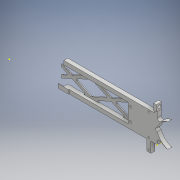
# Autodesk Inventor part: mtv_frame(BrakeInFront)2-6
Saved by Autodesk Inventor 2018 (Build 220112000, 112)
## iProperties
Created: 2019-01-13
Part Number: mtv_frame(BrakeInFront)2-6
Material: Generic
Document SubType Name: Modeling
Designer: aditya
Density: 1 g/cm^3
Appearance: Default
Author: aditya
## iProperties of the stored document mtv_frame(BrakeInFront)1-18 - FRONT_3DPrint.ipt
Created: 2019-01-19
Part Number: mtv_frame(BrakeInFront)1-18 - FRONT_3DPrint
Material: Generic
Document SubType Name: Modeling
Designer: aditya
Density: 1 g/cm^3
Appearance: Default
Author: aditya
Autodesk Inventor part; units mm, degrees
ref_plane "YZ Plane" through (0, 0, 0) normal (1, 0, 0) x (0, 1, 0)
ref_plane "XZ Plane" through (0, 0, 0) normal (0, 1, 0) x (-1, 0, 0)
ref_plane "XY Plane" through (0, 0, 0) normal (0, 0, 1) x (1, 0, 0)
sketch "Sketch1" plane through (0, 0, 0) normal (0, 1, 0) x (-1, 0, 0)
  line L0 (0, 0) -> (50, 0)
  line L1 (50, 0) -> (50, 50)
  line L2 (50, 50) -> (0, 50)
  line L3 (0, 50) -> (0, 0)
  line L4 (50, 50) -> (290, 50)
  line L5 (290, 50) -> (290, 42.5)
  line L6 (290, 42.5) -> (50, 42.5)
  line L7 (50, 42.5) -> (50, 50)
  line L8 (50, 0) -> (290, 0)
  line L9 (290, 0) -> (290, 7.5)
  line L10 (290, 7.5) -> (50, 7.5)
  line L11 (50, 7.5) -> (50, 0)
  dimension "d0" = 50
  dimension "d1" = 50
  dimension "d2" = 240
  dimension "d3" = 7.5
  dimension "d4" = 7.5
  constraints: 24 end point, 6 parallel, 3 horizontal, 3 perpendicular, 1 point on line
  measures "d0" distance of L2.end L1.end
  measures "d1" distance of L1.end L0.end
  measures "d2" distance of L5.end L6.end
  measures "d3" distance of L4.end L5.end
  measures "d4" distance of L9.end L8.end
extrude "Extrusion1" add sketch "Sketch1" along normal blind 7.5
sketch "Sketch2" plane through (0, 7.5, 0) normal (0, 1, 0) x (1, 0, 0)
  line L0 (0, -50) -> (0, 0) projected
  point P0 (0, -25)
  constraints: 1 midpoint
hole "Hole1" at (0, 7.5, 25) direction (0, -1, 0) diameter 6.35 end through all
sketch "Sketch3" plane through (0, 7.5, 0) normal (0, 1, 0) x (1, 0, 0)
  line L0 (-3.175, -50) -> (-3.175, 0) construction
  line L1 (-3.175, -50) -> (-28.175, -50) construction
  line L2 (-28.175, -50) -> (-28.175, 0) construction
  line L3 (-28.175, 0) -> (-3.175, 0) construction
  point P0 (0, 0)
  point P1 (-7.175, -4)
  point P2 (-24.175, -46)
  dimension "d14" = 25
  constraints: 8 end point, 2 perpendicular, 1 vertical
  measures "d14" distance of L0.start L1.end
hole "Hole2" at (-7.175, 7.5, 4) at (-24.175, 7.5, 46) direction (0, -1, 0) diameter 3.3 end through all
sketch "Sketch4" plane through (0, 7.5, 0) normal (0, 1, 0) x (1, 0, 0)
  arc A0 (0, -21.825) -> (0, -28.175) centre (0, -25) ccw construction
  line L0 (-3.175, -25) -> (-28.175, -25) construction
  line L1 (-3.175, -25) -> (21.825, -25) construction
  line L2 (-290, -50) -> (0, -50) construction
  line L3 (-28.175, -50) -> (-28.175, 0) construction
  line L4 (-50, -7.5) -> (-50, -42.5) construction
  line L5 (-50, -42.5) -> (-45, -42.5) construction
  line L6 (-45, -42.5) -> (-45, -32.5) construction
  line L7 (-45, -32.5) -> (-50, -32.5) construction
  line L8 (-50, -32.5) -> (-50, -42.5) construction
  line L9 (-45, -32.5) -> (-40, -32.5)
  line L10 (-40, -32.5) -> (-40, -42.5)
  line L11 (-40, -42.5) -> (-45, -42.5)
  line L12 (-45, -42.5) -> (-45, -32.5)
  point P0 (0, 0)
  dimension "d22" = 25
  dimension "d23" = 180
  dimension "d24" = 5
  dimension "d25" = 10
  dimension "d26" = 5
  constraints: 22 end point, 4 horizontal, 4 parallel, 2 perpendicular, 2 point on line, 1 collinear, 1 point on circle, 1 vertical
  measures "d22" distance of L0.start L0.end
  measures "d23" angle of L0 L1
  measures "d24" distance of L7.end L6.end
  measures "d25" distance of L6.end L5.end
  measures "d26" distance of L10.end L11.end
extrude "Extrusion2" add sketch "Sketch4" along normal blind 17.5
sketch "Sketch5" plane through (0, 7.5, 0) normal (0, 1, 0) x (1, 0, 0)
  line L0 (-85, -7.5) -> (-85, -42.5)
  line L1 (-127.5, -7.5) -> (-127.5, -42.5)
  line L2 (-92.5, -42.5) -> (-92.5, -7.5)
  line L3 (-135, -7.5) -> (-170, -7.5) construction
  line L4 (-170, -7.5) -> (-170, -42.5) construction
  line L5 (-170, -42.5) -> (-135, -42.5) construction
  line L6 (-135, -42.5) -> (-135, -7.5) construction
  line L7 (-177.5, -7.5) -> (-212.5, -7.5) construction
  line L8 (-212.5, -7.5) -> (-212.5, -42.5) construction
  line L9 (-212.5, -42.5) -> (-177.5, -42.5) construction
  line L10 (-177.5, -42.5) -> (-177.5, -7.5) construction
  line L11 (-220, -7.5) -> (-255, -7.5) construction
  line L12 (-255, -7.5) -> (-255, -42.5) construction
  line L13 (-255, -42.5) -> (-220, -42.5) construction
  line L14 (-220, -42.5) -> (-220, -7.5) construction
  line L15 (-85, -7.5) -> (-92.5, -7.5) construction
  line L16 (-92.5, -7.5) -> (-92.5, -42.5) construction
  line L17 (-92.5, -42.5) -> (-85, -42.5) construction
  line L18 (-85, -42.5) -> (-85, -7.5) construction
  line L19 (-127.5, -7.5) -> (-135, -7.5) construction
  line L20 (-135, -7.5) -> (-135, -42.5) construction
  line L21 (-135, -42.5) -> (-127.5, -42.5) construction
  line L22 (-127.5, -42.5) -> (-127.5, -7.5) construction
  line L23 (-170, -7.5) -> (-177.5, -7.5) construction
  line L24 (-177.5, -7.5) -> (-177.5, -42.5) construction
  line L25 (-177.5, -42.5) -> (-170, -42.5) construction
  line L26 (-170, -42.5) -> (-170, -7.5) construction
  line L27 (-212.5, -7.5) -> (-220, -7.5) construction
  line L28 (-220, -7.5) -> (-220, -42.5) construction
  line L29 (-220, -42.5) -> (-212.5, -42.5) construction
  line L30 (-212.5, -42.5) -> (-212.5, -7.5) construction
  line L31 (-220, -7.5) -> (-212.5, -7.5)
  line L32 (-212.5, -7.5) -> (-212.5, -42.5)
  line L33 (-212.5, -42.5) -> (-220, -42.5)
  line L34 (-220, -42.5) -> (-220, -7.5)
  line L35 (-177.5, -7.5) -> (-170, -7.5)
  line L36 (-170, -7.5) -> (-170, -42.5)
  line L37 (-170, -42.5) -> (-177.5, -42.5)
  line L38 (-177.5, -42.5) -> (-177.5, -7.5)
  line L39 (-135, -7.5) -> (-127.5, -7.5)
  line L40 (-127.5, -7.5) -> (-127.5, -42.5)
  line L41 (-127.5, -42.5) -> (-135, -42.5)
  line L42 (-135, -42.5) -> (-135, -7.5)
  line L43 (-92.5, -7.5) -> (-85, -7.5)
  line L44 (-85, -7.5) -> (-85, -42.5)
  line L45 (-85, -42.5) -> (-92.5, -42.5)
  line L46 (-92.5, -42.5) -> (-92.5, -7.5)
  point P0 (0, 0)
  point P1 (-50, -7.5)
  dimension "d30" = 35
  dimension "d31" = 35
  dimension "d32" = 35
  dimension "d33" = 35
  dimension "d34" = 35
  dimension "d35" = 35
  constraints: 94 end point, 23 parallel, 11 horizontal, 11 perpendicular
  measures "d30" distance of L2.start L1.end
  measures "d31" distance of L5.end L4.end
  measures "d32" distance of L4.end L3.end
  measures "d33" distance of L9.end L8.end
  measures "d34" distance of L8.end L7.end
  measures "d35" distance of L13.end L12.end
extrude "Extrusion3" add sketch "Sketch5" against normal blind 2
sketch "Sketch6" plane through (0, 7.5, 0) normal (0, 1, 0) x (1, 0, 0)
  line L0 (-290, 0) -> (-290, -7.5) projected
  line L1 (-290, -50) -> (0, -50) projected
  line L2 (-290, 0) -> (-280, 0)
  line L3 (-280, 0) -> (-280, -50)
  line L4 (-280, -50) -> (-290, -50)
  line L5 (-290, -50) -> (-290, 0)
  point P0 (0, 0)
  dimension "d38" = 10
  constraints: 8 end point, 2 parallel, 1 horizontal, 1 perpendicular, 1 point on line
  measures "d38" distance of L3.end L4.end
extrude "Extrusion4" cut sketch "Sketch6" against normal blind 7.5
sketch "Sketch7" plane through (-280, 7.5, 0) normal (-1, 0, 0) x (0, 0, 1)
  point P0 (0, -7.5)
sketch "Sketch8" plane through (-280, 7.5, 0) normal (-1, 0, 0) x (0, 0, 1)
  line L0 (-25, 0) -> (75, 0)
  line L1 (75, 0) -> (75, -7.5)
  line L2 (75, -7.5) -> (-25, -7.5)
  line L3 (-25, -7.5) -> (-25, 0)
  line L4 (-25, 0) -> (75, 0)
  line L5 (75, 0) -> (75, -10)
  line L6 (75, -10) -> (-25, -10)
  line L7 (-25, -10) -> (-25, 0)
  point P0 (0, -7.5)
  dimension "d41" = 100
  dimension "d42" = 10
  constraints: 16 end point, 4 parallel, 2 horizontal, 2 perpendicular
  measures "d41" distance of L1.end L2.end
  measures "d42" distance of L4.end L5.end
extrude "Extrusion5" add sketch "Sketch8" along normal blind 7.5
sketch "Sketch9" plane through (-287.5, 7.5, 0) normal (-1, 0, 0) x (0, 0, 1)
  line L0 (75, 0) -> (-25, 0) projected
  line L1 (-25, -10) -> (75, -10) projected
  line L2 (-25, 0) -> (-17.5, 0)
  line L3 (-17.5, 0) -> (-17.5, -10)
  line L4 (-17.5, -10) -> (-25, -10)
  line L5 (-25, -10) -> (-25, 0)
  line L6 (75, 0) -> (67.5, 0)
  line L7 (67.5, 0) -> (67.5, -10)
  line L8 (67.5, -10) -> (75, -10)
  line L9 (75, -10) -> (75, 0)
  point P0 (0, -7.5)
  dimension "d45" = 7.5
  dimension "d46" = 7.5
  constraints: 16 end point, 4 parallel, 2 horizontal, 2 perpendicular, 2 point on line
  measures "d45" distance of L3.end L4.end
  measures "d46" distance of L8.end L7.end
extrude "Extrusion6" add sketch "Sketch9" along normal blind 25 contours L9 L1 L7 L0 | L3 L1 L5 L0
sketch "Sketch10" plane through (-287.5, -2.5, -17.5) normal (0, 0, 1) x (1, 0, 0)
  line L0 (0, 0) -> (-25, 0) construction
  line L1 (0, 0) -> (-3, 0) construction
  line L2 (-3, 0) -> (-6.2, 0)
  line L3 (-6.2, 0) -> (-6.2, 2.1)
  line L4 (-6.2, 2.1) -> (-3, 2.1)
  line L5 (-3, 2.1) -> (-3, 0)
  line L6 (-6.2, 2.1) -> (-11.7, 2.1) construction
  line L7 (-11.7, 2.1) -> (-11.7, 5.4) construction
  point P0 (287.5, 2.5)
  dimension "d49" = 3
  dimension "d50" = 3.2
  dimension "d51" = 2.1
  dimension "d52" = 5.5
  dimension "d53" = 3.3
  constraints: 14 end point, 3 perpendicular, 2 point on line, 1 coincident, 1 horizontal, 1 vertical
  measures "d49" distance of L0.start L1.end
  measures "d50" distance of L1.end L2.end
  measures "d51" distance of L2.end L3.end
  measures "d52" distance of L3.end L6.end
  measures "d53" distance of L6.end L7.end
extrude "Extrusion7" add sketch "Sketch10" along normal blind 92.5
sketch "Sketch11" plane through (-287.5, -2.5, -17.5) normal (0, 0, 1) x (1, 0, 0)
  line L0 (-6.2, 2.1) -> (-3, 2.1) construction
  line L1 (-6.2, 2.1) -> (-11.7, 2.1) construction
  line L2 (-11.7, 2.1) -> (-11.7, 5.4) construction
  circle A0 centre (-11.7, 5.4) radius 2.125
  point P0 (287.5, 2.5)
  dimension "d56" = 5.5
  dimension "d57" = 3.3
  dimension "d58" = 4.25
  constraints: 4 end point, 1 centre point, 1 coincident, 1 horizontal, 1 perpendicular
  measures "d56" distance of L0.start L1.end
  measures "d57" distance of L1.end L2.end
  measures "d58" diameter of A0
extrude "Extrusion8" cut sketch "Sketch11" along normal mid plane 241
sketch "Sketch12" plane through (-287.5, -2.5, -17.5) normal (0, 0, 1) x (1, 0, 0)
  circle A0 centre (-11.7, 5.4) radius 2.125 construction
  line L0 (-11.7, 5.4) -> (-11.7, 0.96) construction
  line L1 (-11.7, 0.96) -> (-16.7, 0.96) construction
  line L2 (-6.2, 0) -> (-25, 0) projected
  line L3 (-16.7, 0.96) -> (-19.2, 0.96)
  line L4 (-19.2, 0.96) -> (-19.2, 0)
  line L5 (-19.2, 0) -> (-16.7, 0)
  line L6 (-16.7, 0) -> (-16.7, 0.96)
  point P0 (287.5, 2.5)
  dimension "d61" = 4.44
  dimension "d62" = 5
  dimension "d63" = 2.5
  constraints: 12 end point, 2 parallel, 2 perpendicular, 1 coincident, 1 horizontal, 1 point on line, 1 vertical
  measures "d61" distance of L0.start L0.end
  measures "d62" distance of L0.end L1.end
  measures "d63" distance of L5.end L4.end
extrude "Extrusion9" add sketch "Sketch12" along normal blind 91.25
sketch "Sketch13" plane through (-293.7, -0.4, -17.5) normal (0, 1, 0) x (1, 0, 0)
  line L0 (3.2, 0) -> (3.2, -85) construction
  line L1 (3.2, 0) -> (3.2, -30) construction
  line L2 (0, 0) -> (0, -85) construction
  line L3 (3.2, -30) -> (0, -30) construction
  line L4 (0, -30) -> (0, -36.35) construction
  line L5 (0, -36.35) -> (3.2, -36.35) construction
  line L6 (3.2, -36.35) -> (3.2, -30) construction
  line L7 (0, -30) -> (3.2, -30)
  line L8 (3.2, -30) -> (3.2, -36.35)
  line L9 (3.2, -36.35) -> (0, -36.35)
  line L10 (0, -36.35) -> (0, -30)
  point P0 (293.7, -17.5)
  dimension "d66" = 30
  dimension "d67" = 6.35
  constraints: 18 end point, 4 parallel, 2 horizontal, 2 perpendicular, 2 point on line
  measures "d66" distance of L0.start L1.end
  measures "d67" distance of L4.end L3.end
extrude "Extrusion10" add sketch "Sketch13" along normal blind 3.8
sketch "Sketch14" plane through (0, 7.5, 0) normal (0, 1, 0) x (1, 0, 0)
  line L0 (-287.5, 17.5) -> (-287.5, -67.5) projected
  line L1 (-287.5, 17.5) -> (-285, 17.5)
  line L2 (-285, 17.5) -> (-285, -67.5)
  line L3 (-285, -67.5) -> (-287.5, -67.5)
  line L4 (-287.5, -67.5) -> (-287.5, 17.5)
  point P0 (0, 0)
  dimension "d70" = 2.5
  constraints: 8 end point, 2 parallel, 1 horizontal, 1 perpendicular
  measures "d70" distance of L2.end L3.end
extrude "Extrusion11" cut sketch "Sketch14" against normal blind 14.55
sketch "Sketch15" plane through (0, 7.5, 0) normal (0, 1, 0) x (1, 0, 0)
  line L0 (-312.5, 17.5) -> (-312.5, 25) projected
  line L1 (-280, -75) -> (-312.5, -75) projected
  line L2 (-312.5, 25) -> (-306.6488, 25)
  line L3 (-306.6488, 25) -> (-306.6488, -75)
  line L4 (-306.6488, -75) -> (-312.5, -75)
  line L5 (-312.5, -75) -> (-312.5, 25)
  point P0 (0, 0)
  constraints: 8 end point, 2 parallel, 1 horizontal, 1 perpendicular, 1 point on line
extrude "Extrusion12" cut sketch "Sketch15" against normal blind 14.55
fillet "Fillet1" radius 0.1 1 edges at (-301.325, 2.9, -17.5)
fillet "Fillet2" radius 0.1 1 edges at (-301.325, 2.9, 67.5)
fillet "Fillet3" radius 3.25 1 edges at (-280, 2.5, 75)
fillet "Fillet4" radius 3.25 1 edges at (-285, 2.5, 67.5)
fillet "Fillet5" radius 3.25 1 edges at (-280, 2.5, -25)
fillet "Fillet6" radius 3.25 1 edges at (-285, 2.5, -17.5)
sketch "Sketch16" plane through (0, 7.5, 0) normal (0, 1, 0) x (1, 0, 0)
  line L0 (-220, -42.5) -> (-220, -7.5) construction
  line L1 (-220, -42.5) -> (-280, -42.5) construction
  line L2 (-220, -7.5) -> (-255, -7.5) construction
  line L3 (-255, -7.5) -> (-255, -42.5) construction
  line L4 (-255, -42.5) -> (-220, -42.5) construction
  line L5 (-220, -42.5) -> (-220, -7.5) construction
  line L6 (-280, -7.5) -> (-280, 0) projected
  line L7 (-280, -7.5) -> (-270, -7.5)
  line L8 (-270, -7.5) -> (-270, -42.5)
  line L9 (-270, -42.5) -> (-280, -42.5)
  line L10 (-280, -42.5) -> (-280, -7.5)
  point P0 (0, 0)
  dimension "d81" = 35
  dimension "d82" = 10
  constraints: 16 end point, 4 parallel, 2 horizontal, 2 perpendicular, 2 point on line
  measures "d81" distance of L4.end L3.end
  measures "d82" distance of L8.end L9.end
extrude "Extrusion13" add sketch "Sketch16" against normal blind 2
sketch "Sketch17" plane through (0, 7.5, 0) normal (0, 1, 0) x (1, 0, 0)
  point P0 (0, 0)
sketch "Sketch18" plane through (0, 7.5, 0) normal (0, 1, 0) x (1, 0, 0)
  line L0 (-270, -7.5) -> (-270, -42.5) construction
  line L1 (-285, -64.25) -> (-285, 14.25) construction
  line L2 (-280, -7.5) -> (-280, 0) construction
  line L3 (-270, -7.5) -> (-280, -7.5) construction
  line L4 (-275, -7.5) -> (-275, -42.5) construction
  line L5 (-50, -42.5) -> (-280, -42.5) construction
  circle A0 centre (-275, -12.5) radius 1.8 construction
  circle A1 centre (-275, -37.5) radius 1.8 construction
  circle A2 centre (-275, -12.5) radius 1.8
  circle A3 centre (-275, -37.5) radius 1.8
  point P0 (0, 0)
  dimension "d85" = 3.6
  dimension "d86" = 3.6
  constraints: 4 centre point, 4 end point, 3 point on line, 2 coincident, 2 concentric, 1 horizontal, 1 midpoint, 1 vertical
  measures "d85" diameter of A0
  measures "d86" diameter of A1
hole "Hole3" at (-275, 7.5, 12.5) at (-275, 7.5, 37.5) direction (0, -1, 0) diameter 3.3 depth 15 tip angle 118
sketch "Sketch19" plane through (0, 7.5, 0) normal (0, 1, 0) x (1, 0, 0)
  circle A0 centre (-275, -12.5) radius 1.65 construction
  line L0 (-275, -12.5) -> (-212.5, -12.5) construction
  line L1 (-212.5, -7.5) -> (-212.5, -42.5) construction
  circle A1 centre (-275, -37.5) radius 1.65 construction
  line L2 (-275, -37.5) -> (-212.5, -37.5) construction
  line L3 (-220, -42.5) -> (-220, -7.5) construction
  line L4 (-220, -12.5) -> (-212.5, -12.5) construction
  line L5 (-216.25, -12.5) -> (-216.25, -37.5) construction
  point P0 (0, 0)
  constraints: 8 end point, 4 point on line, 3 horizontal, 2 coincident, 1 midpoint, 1 perpendicular
hole "Hole4" at (-216.25, 7.5, 12.5) at (-216.25, 7.5, 37.5) direction (0, -1, 0) diameter 3.3 depth 15 tip angle 118
sketch "Sketch20" plane through (-45, 7.5, 32.5) normal (-1, 0, 0) x (0, 0, 1)
  line L0 (10, 17.5) -> (0, 17.5) construction
  line L1 (5, 17.5) -> (5, -0.1335) construction
  line L2 (10, 0) -> (10, 17.5) construction
  line L3 (10, 12.5) -> (5, 12.5) construction
  circle A0 centre (5, 12.5) radius 3
  point P0 (-32.5, -7.5)
  dimension "d101" = 6
  constraints: 4 end point, 2 coincident, 2 point on line, 1 centre point, 1 midpoint, 1 perpendicular, 1 vertical
  measures "d101" diameter of A0
extrude "Extrusion14" cut sketch "Sketch20" against normal blind 20
sketch "Sketch21" plane through (0, 7.5, 0) normal (0, 1, 0) x (1, 0, 0)
  line L0 (-306.6488, 17.5) -> (-306.6488, -67.5) projected
  line L1 (-306.6488, 17.5) -> (-288.25, 17.5) projected
  line L2 (-306.6488, -67.5) -> (-288.25, -67.5)
  line L3 (-288.25, -67.5) -> (-288.25, 17.5)
  line L4 (-288.25, 17.5) -> (-306.6488, 17.5)
  line L5 (-306.6488, 17.5) -> (-306.6488, -67.5)
  point P0 (0, 0)
  constraints: 8 end point, 2 parallel, 1 horizontal, 1 perpendicular
extrude "Extrusion15" cut sketch "Sketch21" against normal blind 10
sketch "Sketch22" plane through (0, 7.5, 0) normal (0, 1, 0) x (1, 0, 0)
  line L0 (-280, -50) -> (0, -50) projected
  line L1 (0, 0) -> (-280, 0) projected
  line L2 (-280, -50) -> (-270.5687, -50)
  line L3 (-270.5687, -50) -> (-270.5687, 0)
  line L4 (-270.5687, 0) -> (-280, 0)
  line L5 (-280, 0) -> (-280, -50)
  line L6 (-50, -42.5) -> (-280, -42.5) projected
  line L7 (-219.3019, -42.5) -> (-213.3073, -42.5)
  line L8 (-213.3073, -42.5) -> (-213.3073, -8.284)
  line L9 (-213.3073, -8.284) -> (-219.3019, -8.284)
  line L10 (-219.3019, -8.284) -> (-219.3019, -42.5)
  constraints: 16 end point, 4 parallel, 2 horizontal, 2 perpendicular, 2 point on line
extrude "Extrusion16" add sketch "Sketch22" against normal blind 2
sketch "Sketch23" plane through (-306.6488, -2.5, -25) normal (0, 0, -1) x (-1, 0, 0)
  circle A0 centre (-7.4488, 5.4) radius 2.125 projected
  circle A1 centre (-7.4488, 5.4) radius 2
  circle A2 centre (-7.4488, 5.4) radius 2.4429
  point P0 (-306.6488, 2.5)
  dimension "d108" = 4
  constraints: 2 centre point, 2 coincident
  measures "d108" diameter of A1
extrude "Extrusion17" add sketch "Sketch23" against normal blind 100 contours A0 | A2
sketch "Sketch24" plane through (0, 7.5, 0) normal (0, 1, 0) x (1, 0, 0)
  line L0 (-288.25, -67.5) -> (-306.6488, -67.5) projected
  arc A0 (-285, 14.25) -> (-288.25, 17.5) centre (-288.25, 14.25) ccw projected
  line L1 (-306.6488, -67.5) -> (-288.25, -67.5)
  line L2 (-288.25, -67.5) -> (-288.25, 17.5)
  line L3 (-288.25, 17.5) -> (-306.6488, 17.5)
  line L4 (-306.6488, 17.5) -> (-306.6488, -67.5)
  point P0 (0, 0)
  constraints: 8 end point, 2 parallel, 1 horizontal, 1 perpendicular
extrude "Extrusion18" cut sketch "Sketch24" against normal blind 100
sketch "Sketch25" plane through (0, 7.5, 0) normal (0, 1, 0) x (1, 0, 0)
  line L0 (-50, -42.5) -> (-280, -42.5) projected
  line L1 (-280, -7.5) -> (-50, -7.5) projected
  line L2 (-50, -42.5) -> (-55, -42.5)
  line L3 (-55, -42.5) -> (-55, -7.5)
  line L4 (-55, -7.5) -> (-50, -7.5)
  line L5 (-50, -7.5) -> (-50, -42.5)
  point P0 (0, 0)
  dimension "d113" = 5
  constraints: 8 end point, 2 parallel, 1 horizontal, 1 perpendicular, 1 point on line
  measures "d113" distance of L3.end L4.end
extrude "Extrusion19" add sketch "Sketch25" against normal blind 2
sketch "Sketch26" plane through (0, 7.5, 0) normal (0, 1, 0) x (1, 0, 0)
  line L0 (-55, -42.5) -> (-85, -42.5) construction
  line L1 (-55, -42.5) -> (-50, -42.5) construction
  line L2 (-55, -42.5) -> (-50, -42.5) construction
  line L3 (-50, -42.5) -> (-50, -7.5) construction
  line L4 (-50, -42.5) -> (-50, -7.5) construction
  circle A0 centre (-50, -37.5) radius 1.65 construction
  circle A1 centre (-50, -12.5) radius 1.65 construction
  circle A2 centre (-50, -37.5) radius 1.65
  circle A3 centre (-50, -12.5) radius 1.65
  line L5 (-50, -37.5) -> (-92.5, -37.5) construction
  line L6 (-92.5, -42.5) -> (-92.5, -7.5) construction
  line L7 (-50, -12.5) -> (-92.5, -12.5) construction
  line L8 (-92.5, -37.5) -> (-85, -37.5) construction
  line L9 (-85, -7.5) -> (-85, -42.5) construction
  line L10 (-88.75, -37.5) -> (-88.75, -12.5) construction
  circle A4 centre (-88.75, -37.5) radius 1.65
  circle A5 centre (-88.75, -12.5) radius 1.65
  point P0 (0, 0)
  dimension "d116" = 3.3
  dimension "d117" = 3.3
  dimension "d118" = 3.3
  dimension "d119" = 3.3
  constraints: 12 end point, 6 centre point, 5 point on line, 4 coincident, 2 concentric, 2 horizontal, 2 perpendicular, 1 collinear, 1 midpoint
  measures "d116" diameter of A0
  measures "d117" diameter of A1
  measures "d118" diameter of A4
  measures "d119" diameter of A5
extrude "Extrusion20" cut sketch "Sketch26" against normal blind 2
sketch "Sketch27" plane through (0, 5.5, 0) normal (0, -1, 0) x (1, 0, 0)
  line L0 (-50, 7.5) -> (-55, 7.5) projected
  line L1 (-55, 7.5) -> (-46.6169, 7.5)
  line L2 (-46.6169, 7.5) -> (-46.6169, 42.5)
  line L3 (-46.6169, 42.5) -> (-55, 42.5)
  line L4 (-55, 42.5) -> (-55, 7.5)
  point P0 (0, 0)
  constraints: 8 end point, 2 parallel, 1 horizontal, 1 perpendicular
extrude "Extrusion21" add sketch "Sketch27" along normal blind 5.5
sketch "Sketch28" plane through (0, 7.5, 0) normal (0, 1, 0) x (1, 0, 0)
  circle A0 centre (-50, -12.5) radius 1.65 projected
  circle A1 centre (-50, -37.5) radius 1.65 projected
  point P0 (0, 0)
  constraints: 2 coincident
hole "Hole5" at (-50, 7.5, 12.5) at (-50, 7.5, 37.5) direction (0, -1, 0) diameter 3.3 depth 8 tip angle 118
sketch "Sketch29" plane through (0, 7.5, 0) normal (0, 1, 0) x (1, 0, 0)
  circle A0 centre (-7.175, -4) radius 1.65 construction
  circle A1 centre (-24.175, -46) radius 1.65 construction
  line L0 (-7.175, -4) -> (-24.175, -46) construction
  line L1 (-7.175, -4) -> (-7.175, -46) construction
  line L2 (-7.175, -46) -> (-24.175, -46) construction
  line L3 (-7.175, -25) -> (-25.825, -25) construction
  line L4 (-25.825, -25) -> (-25.825, -46) construction
  line L5 (-16.5, -25) -> (-25.825, -25) construction
  line L6 (-24.175, -46) -> (-24.175, -25) construction
  line L7 (-15.675, -46) -> (-15.675, -4) construction
  line L8 (-40, -32.5) -> (-40, -42.5) construction
  line L9 (-40, -42.5) -> (-24.175, -42.5) construction
  line L10 (-24.175, -42.5) -> (-24.175, -46) construction
  line L11 (-15.675, -25) -> (-15.675, -46) construction
  line L12 (-15.675, -46) -> (-15.675, -4) construction
  circle A2 centre (-15.675, -46) radius 1.65 construction
  circle A3 centre (-15.675, -46) radius 1.65
  circle A4 centre (-15.675, -4) radius 1.65
  point P0 (0, 0)
  dimension "d131" = 42
  dimension "d132" = 17
  dimension "d133" = 21
  dimension "d135" = 8.5
  dimension "d136" = 15.825
  dimension "d137" = 3.5
  dimension "d138" = 21
  dimension "d139" = 3.3
  dimension "d140" = 3.3
  dimension "d141" = 3.3
  constraints: 24 end point, 4 collinear, 4 midpoint, 4 perpendicular, 3 centre point, 3 coincident, 3 point on line, 2 vertical, 1 horizontal, 1 horizontal alignment, 1 other
  measures "d131" distance of L0.start L1.end
  measures "d132" distance of L1.end L2.end
  measures "d133" distance of L3.end L4.end
  measures "d135" distance of L11.start L3.start
  measures "d136" distance of L8.end L9.end
  measures "d137" distance of L9.end L2.end
  measures "d138" distance of L11.start L7.start
  measures "d139" diameter of A2
  measures "d140" diameter of A3
  measures "d141" diameter of A4
extrude "Extrusion22" cut sketch "Sketch29" against normal blind 10
sketch "Sketch30" plane through (0, 7.5, 0) normal (0, 1, 0) x (1, 0, 0)
  circle A0 centre (-7.175, -4) radius 1.65 projected
  circle A1 centre (-7.175, -4) radius 2.1021
  circle A2 centre (-24.175, -46) radius 1.65 projected
  circle A3 centre (-24.175, -46) radius 2.9173
  point P0 (0, 0)
  constraints: 2 centre point, 2 coincident
extrude "Extrusion23" add sketch "Sketch30" against normal blind 7.5 contours A0 | A1 | A2 | A3
sketch "Sketch31" plane through (0, 7.5, 0) normal (0, 1, 0) x (1, 0, 0)
  line L0 (-45, -42.5) -> (-45, -32.5) construction
  circle A0 centre (-50, -37.5) radius 1.65 construction
  line L1 (-45, -37.5) -> (-50, -37.5) construction
  circle A1 centre (-50, -12.5) radius 1.65 construction
  line L2 (-50, -12.5) -> (-45, -12.5) construction
  line L3 (-40, -32.5) -> (-40, -42.5) construction
  line L4 (-40, -42.5) -> (-45, -32.5) construction
  line L5 (-45, -32.5) -> (-40, -32.5) construction
  line L6 (-40, -32.5) -> (-45, -42.5) construction
  line L7 (-50, -37.5) -> (-42.5, -37.5) construction
  line L8 (-42.5, -37.5) -> (-42.5, -12.5) construction
  line L9 (-45, -17.5) -> (-40, -17.5)
  line L10 (-40, -17.5) -> (-40, -7.5)
  line L11 (-40, -7.5) -> (-45, -7.5)
  line L12 (-45, -7.5) -> (-45, -17.5)
  line L13 (-45, -17.5) -> (-40, -7.5) construction
  line L14 (-40, -17.5) -> (-45, -7.5) construction
  point P0 (0, 0)
  dimension "d146" = 5
  dimension "d147" = 10
  dimension "d148" = 5
  dimension "d149" = 10
  constraints: 24 end point, 5 midpoint, 3 horizontal, 2 parallel, 1 perpendicular, 1 vertical
  measures "d146" distance of L1.start L1.end
  measures "d147" distance of L3.start L3.end
  measures "d148" distance of L11.end L10.end
  measures "d149" distance of L10.end L9.end
extrude "Extrusion24" add sketch "Sketch31" along normal blind 17.5
sketch "Sketch32" plane through (-45, 7.5, 7.5) normal (-1, 0, 0) x (0, 0, 1)
  line L0 (10, 17.5) -> (0, 17.5) construction
  line L1 (5, 17.5) -> (5, 12.5) construction
  point P0 (-7.5, -7.5)
  dimension "d152" = 5
  constraints: 2 end point, 1 midpoint, 1 vertical
  measures "d152" distance of L1.start L1.end
hole "Hole6" at (-45, 20, 12.5) direction (1, 0, 0) diameter 7 depth 8 tip angle 118
sketch "Sketch33" plane through (0, 25, 0) normal (0, 1, 0) x (1, 0, 0)
  line L0 (-45, -32.5) -> (-40, -32.5) projected
  line L1 (-40, -32.5) -> (-40, -42.5) projected
  line L2 (-45, -32.5) -> (-40, -32.5)
  line L3 (-40, -32.5) -> (-40, -42.5)
  line L4 (-40, -42.5) -> (-45, -42.5)
  line L5 (-45, -42.5) -> (-45, -32.5)
  point P0 (0, 0)
  constraints: 8 end point, 2 parallel, 1 horizontal, 1 perpendicular
extrude "Extrusion25" cut sketch "Sketch33" against normal blind 17.5
sketch "Sketch34" plane through (0, 7.5, 0) normal (0, 1, 0) x (1, 0, 0)
  line L0 (-280, -50) -> (0, -50) projected
  line L1 (-176.6721, -50) -> (-309.3974, -50)
  line L2 (-309.3974, -50) -> (-309.3974, 41.697)
  line L3 (-309.3974, 41.697) -> (-176.6721, 41.697)
  line L4 (-176.6721, 41.697) -> (-176.6721, -50)
  line L5 (-176.6721, 41.697) -> (-320.285, 41.697)
  line L6 (-320.285, 41.697) -> (-320.285, -112.2851)
  line L7 (-320.285, -112.2851) -> (-176.6721, -112.2851)
  line L8 (-176.6721, -112.2851) -> (-176.6721, 41.697)
  point P0 (0, 0)
  constraints: 16 end point, 4 parallel, 2 horizontal, 2 perpendicular, 1 point on line
extrude "Extrusion26" cut sketch "Sketch34" against normal blind 170.5
sketch "Sketch35" plane through (-176.6721, 7.5, 0) normal (-1, 0, 0) x (0, 0, 1)
  line L0 (42.5, -7.5) -> (7.5, -7.5) construction
  line L1 (0, 0) -> (7.5, -7.5) construction
  line L2 (7.5, -7.5) -> (7.5, 0) construction
  line L3 (21.825, -7.5) -> (0, -7.5) construction
  line L4 (7.5, 0) -> (0, -7.5) construction
  line L5 (5.625, -5.625) -> (1.875, -5.625)
  line L6 (1.875, -5.625) -> (1.875, -1.875)
  line L7 (1.875, -1.875) -> (5.625, -1.875)
  line L8 (5.625, -1.875) -> (5.625, -5.625)
  line L9 (5.625, -5.625) -> (1.875, -1.875) construction
  line L10 (1.875, -5.625) -> (5.625, -1.875) construction
  line L11 (42.5, -7.5) -> (50, 0) construction
  line L12 (50, 0) -> (50, -7.5) construction
  line L13 (50, -7.5) -> (42.5, 0) construction
  line L14 (0, 0) -> (50, 0) construction
  line L15 (48.125, -5.625) -> (44.375, -5.625)
  line L16 (44.375, -5.625) -> (44.375, -1.875)
  line L17 (44.375, -1.875) -> (48.125, -1.875)
  line L18 (48.125, -1.875) -> (48.125, -5.625)
  line L19 (48.125, -5.625) -> (44.375, -1.875) construction
  line L20 (44.375, -5.625) -> (48.125, -1.875) construction
  point P0 (3.75, -3.75)
  point P1 (46.25, -3.75)
  dimension "d164" = 3.75
  dimension "d165" = 3.75
  dimension "d166" = 3.75
  dimension "d167" = 3.75
  constraints: 36 end point, 6 midpoint, 5 perpendicular, 4 parallel, 2 horizontal, 1 point on line, 1 vertical
  measures "d164" distance of L6.end L7.end
  measures "d165" distance of L5.end L6.end
  measures "d166" distance of L16.end L17.end
  measures "d167" distance of L15.end L16.end
extrude "Extrusion27" add sketch "Sketch35" along normal blind 10
sketch "Sketch36" plane through (-176.6721, 5.625, 48.125) normal (0, 1, 0) x (1, 0, 0)
  line L0 (0, 0) -> (-13.3619, 0)
  line L1 (-13.3619, 0) -> (-13.3619, 48.125)
  line L2 (-13.3619, 48.125) -> (0, 48.125)
  line L3 (0, 48.125) -> (0, 0)
  point P0 (176.6721, 48.125)
  constraints: 8 end point, 2 parallel, 1 horizontal, 1 perpendicular
extrude "Extrusion28" cut sketch "Sketch36" against normal blind 100
sketch "Sketch37" plane through (-176.6721, 7.5, 0) normal (-1, 0, 0) x (0, 0, 1)
  line L0 (42.5, -7.5) -> (42.5, -2) construction
  line L1 (50, 0) -> (28.175, 0) construction
  line L2 (42.5, -7.5) -> (50, 0) construction
  line L3 (50, 0) -> (50, -7.5) construction
  line L4 (50, -7.5) -> (46.25, -3.75) construction
  line L5 (42.5, -7.5) -> (7.5, -7.5) construction
  line L6 (0, -7.5) -> (0, 0) construction
  line L7 (7.5, -7.5) -> (0, 0) construction
  line L8 (21.825, -7.5) -> (0, -7.5) construction
  line L9 (0, 0) -> (0, -7.5) construction
  line L10 (0, -7.5) -> (3.75, -3.75) construction
  constraints: 12 end point, 2 coincident, 2 midpoint, 2 perpendicular, 1 parallel
hole "Hole7" at (-176.6721, 3.75, 46.25) at (-176.6721, 3.75, 3.75) direction (1, 0, 0) diameter 5 depth 15
sketch "Sketch38" plane through (0, 7.5, 0) normal (0, 1, 0) x (1, 0, 0)
  line L0 (-91.4577, -41.6279) -> (-86.1085, -41.6279)
  line L1 (-86.1085, -41.6279) -> (-86.1085, -9.2314)
  line L2 (-86.1085, -9.2314) -> (-91.4577, -9.2314)
  line L3 (-91.4577, -9.2314) -> (-91.4577, -41.6279)
  point P0 (0, 0)
  constraints: 8 end point, 2 parallel, 1 horizontal, 1 perpendicular
extrude "Extrusion29" add sketch "Sketch38" against normal blind 2
sketch "Sketch39" plane through (0, 0, 50) normal (0, 0, 1) x (1, 0, 0)
  line L0 (-176.6721, 7.5) -> (0, 7.5) projected
  line L1 (0, 0) -> (-5, 0)
  line L2 (-5, 0) -> (-5, 7.5)
  line L3 (-5, 7.5) -> (0, 7.5)
  line L4 (0, 7.5) -> (0, 0)
  dimension "d181" = 5
  constraints: 8 end point, 2 parallel, 1 horizontal, 1 perpendicular, 1 point on line
  measures "d181" distance of L2.end L3.end
extrude "Extrusion30" add sketch "Sketch39" along normal blind 15
sketch "Sketch40" plane through (0, 0, 28.175) normal (1, 0, 0) x (0, 0, -1)
  line L0 (0, 0) -> (-36.825, 0) construction
  line L1 (-36.825, 0) -> (-29.325, 0) construction
  line L2 (-21.825, 7.5) -> (-36.825, 7.5) construction
  line L3 (-29.325, 0) -> (-36.825, 7.5) construction
  line L4 (-36.825, 7.5) -> (-36.825, 0) construction
  line L5 (-36.825, 7.5) -> (-36.825, 0) construction
  line L6 (-33.075, 3.75) -> (-36.825, 0) construction
  point P0 (28.175, 0)
  dimension "d184" = 7.5
  constraints: 8 end point, 1 midpoint, 1 perpendicular, 1 point on line
  measures "d184" distance of L0.end L1.end
hole "Hole8" at (0, 3.75, 61.25) direction (-1, 0, 0) diameter 6 depth 15
sketch "Sketch41" plane through (0, 25, 0) normal (0, 1, 0) x (1, 0, 0)
  line L0 (-45, -17.5) -> (-45, -7.5) projected
  line L1 (-40, -7.5) -> (-40, -17.5) projected
  line L2 (-45, -17.5) -> (-40, -17.5)
  line L3 (-40, -17.5) -> (-40, -7.5)
  line L4 (-40, -7.5) -> (-45, -7.5)
  line L5 (-45, -7.5) -> (-45, -17.5)
  point P0 (0, 0)
  constraints: 8 end point, 2 parallel, 1 horizontal, 1 perpendicular
extrude "Extrusion31" cut sketch "Sketch41" against normal blind 17.5
sketch "Sketch42" plane through (0, 7.5, 0) normal (0, 1, 0) x (1, 0, 0)
  arc A0 (0, -21.825) -> (0, -28.175) centre (0, -25) ccw construction
  line L0 (0, -25) -> (0, -1.25) construction
  line L1 (0, -21.825) -> (0, 0) construction
  line L2 (0, -1.25) -> (0, -48.75) construction
  line L3 (0, -28.175) -> (0, -65) construction
  line L4 (0, -25) -> (3.175, -25) construction
  arc A1 (26.925, -1.25) -> (26.925, -48.75) centre (26.925, -25) ccw construction
  line L5 (0, -1.25) -> (20, -1.25) construction
  line L6 (20, -1.25) -> (20, -25) construction
  line L7 (20, -25) -> (20, -48.75) construction
  arc A2 (20, -2.282) -> (0, -21.825) centre (29.1085, -31.6088) ccw
  arc A3 (0, -28.175) -> (20, -47.718) centre (29.6425, -17.8446) ccw
  line L8 (0, -28.175) -> (0, -33.175)
  line L9 (0, -21.825) -> (0, -16.825)
  arc A4 (0, -33.175) -> (20, -47.718) centre (25.4273, -19.2304) ccw
  arc A5 (20, -2.282) -> (0, -16.825) centre (25.4273, -30.7696) ccw
  dimension "d194" = 23.75
  dimension "d195" = 47.5
  dimension "d200" = 20
  dimension "d203" = 5
  dimension "d204" = 5
  dimension "d205" = 29
  dimension "d206" = 29
  constraints: 16 end point, 13 point on circle, 7 point on line, 5 centre point, 2 horizontal, 1 perpendicular
  measures "d194" distance of L0.start L0.end
  measures "d195" distance of L0.end L2.end
  measures "d200" distance of L0.end L5.end
  measures "d203" distance of L3.start L8.end
  measures "d204" distance of L1.start L9.end
  measures "d205" radius of A4
  measures "d206" radius of A5
extrude "Extrusion32" add sketch "Sketch42" against normal blind 7.5
fillet "Fillet7" radius 4 1 edges at (0, 3.75, 33.175)
fillet "Fillet8" radius 4 1 edges at (0, 3.75, 16.825)
sketch "Sketch43" plane through (0, 0, 65) normal (0, 0, 1) x (1, 0, 0)
  line L0 (0, 0) -> (0, 7.5) projected
  line L1 (-5, 0) -> (-5, 7.5) projected
  line L2 (0, 0) -> (-5, 0)
  line L3 (-5, 0) -> (-5, 7.5)
  line L4 (-5, 7.5) -> (0, 7.5)
  line L5 (0, 7.5) -> (0, 0)
  constraints: 8 end point, 2 parallel, 1 horizontal, 1 perpendicular
extrude "Extrusion33" add sketch "Sketch43" along normal blind 2
sketch "Sketch44" plane through (0, 0, 0) normal (0, -1, 0) x (1, 0, 0)
  line L0 (0, 44.3276) -> (0, 67) projected
  line L1 (-5, 50) -> (-5, 67) projected
  line L2 (0, 67) -> (-5, 67)
  line L3 (-5, 67) -> (-5, 55)
  line L4 (-5, 55) -> (0, 55)
  line L5 (0, 55) -> (0, 67)
  point P0 (0, 0)
  dimension "d213" = 12
  constraints: 8 end point, 2 parallel, 1 horizontal, 1 perpendicular, 1 point on line
  measures "d213" distance of L3.end L2.end
extrude "Extrusion34" add sketch "Sketch44" along normal blind 2
sketch "Sketch45" plane through (0, 0, 0) normal (0, 0, -1) x (-1, 0, 0)
  point P0 (0, 0)
sketch "Sketch46" plane through (0, 7.5, 0) normal (0, 1, 0) x (1, 0, 0)
  circle A0 centre (-15.675, -46) radius 1.65 construction
  line L0 (-15.675, -46) -> (-15.675, 0) construction
  point P0 (0, 0)
  constraints: 2 end point, 1 vertical
sketch "Sketch47" plane through (0, 0, 0) normal (0, 0, -1) x (-1, 0, 0)
  line L0 (0, 7.5) -> (176.6721, 7.5) construction
  line L1 (15.675, 7.5) -> (15.675, 0) construction
  line L2 (0, 0) -> (176.6721, 0) construction
  line L3 (19.425, 0) -> (11.925, 0) construction
  line L4 (11.925, 0) -> (11.925, 7.5) construction
  line L5 (11.925, 7.5) -> (19.425, 7.5) construction
  line L6 (19.425, 7.5) -> (19.425, 0) construction
  line L7 (19.425, 0) -> (11.925, 7.5) construction
  line L8 (11.925, 0) -> (19.425, 7.5) construction
  line L9 (19.425, 0) -> (11.925, 0)
  line L10 (11.925, 0) -> (11.925, 7.5)
  line L11 (11.925, 7.5) -> (19.425, 7.5)
  line L12 (19.425, 7.5) -> (19.425, 0)
  line L13 (19.425, 0) -> (11.925, 7.5) construction
  line L14 (11.925, 0) -> (19.425, 7.5) construction
  point P0 (15.675, 3.75)
  point P1 (15.675, 3.75)
  dimension "d216" = 7.5
  dimension "d217" = 7.5
  constraints: 26 end point, 6 midpoint, 4 parallel, 2 horizontal, 2 perpendicular, 2 point on line, 1 vertical
  measures "d216" distance of L4.end L5.end
  measures "d217" distance of L3.end L4.end
extrude "Extrusion35" add sketch "Sketch47" along normal blind 20
sketch "Sketch48" plane through (0, 7.5, 0) normal (0, 1, 0) x (1, 0, 0)
  circle A0 centre (-15.675, -4) radius 1.65 construction
  line L0 (-15.675, -4) -> (-15.675, 16) construction
  circle A1 centre (-15.675, 16) radius 1.65
  point P0 (0, 0)
  dimension "d220" = 20
  dimension "d221" = 3.3
  constraints: 2 end point, 1 centre point, 1 coincident, 1 vertical
  measures "d220" distance of L0.start L0.end
  measures "d221" diameter of A1
extrude "Extrusion36" cut sketch "Sketch48" against normal blind 20
sketch "Sketch49" plane through (0, 7.5, 0) normal (0, 1, 0) x (1, 0, 0)
  circle A0 centre (-50, -37.5) radius 1.65 projected
  circle A1 centre (-50, -37.5) radius 2
  circle A2 centre (-50, -12.5) radius 1.65 projected
  circle A3 centre (-50, -12.5) radius 2
  point P0 (0, 0)
  dimension "d224" = 4
  dimension "d225" = 4
  constraints: 2 centre point, 2 coincident
  measures "d224" diameter of A1
  measures "d225" diameter of A3
extrude "Extrusion37" cut sketch "Sketch49" against normal blind 10 contours A0 | A1 | A3
sketch "Sketch50" plane through (0, 5.5, 0) normal (0, -1, 0) x (1, 0, 0)
  line L0 (-176.6721, 0) -> (-176.6721, 50) construction
  line L1 (-176.6721, 25) -> (-55, 25) construction
  line L2 (-55, 42.5) -> (-55, 7.5) construction
  line L3 (-176.6721, 23.5) -> (-55, 23.5)
  line L4 (-55, 23.5) -> (-55, 26.5)
  line L5 (-55, 26.5) -> (-176.6721, 26.5)
  line L6 (-176.6721, 26.5) -> (-176.6721, 23.5)
  line L7 (-176.6721, 23.5) -> (-55, 26.5) construction
  line L8 (-55, 23.5) -> (-176.6721, 26.5) construction
  point P0 (0, 0)
  point P1 (-115.836, 25)
  dimension "d228" = 3
  constraints: 14 end point, 5 midpoint, 2 parallel, 1 horizontal, 1 perpendicular, 1 point on line
  measures "d228" distance of L4.end L3.end
extrude "Extrusion38" add sketch "Sketch50" along normal blind 5.5
sketch "Sketch51" plane through (0, 7.5, 0) normal (0, 1, 0) x (1, 0, 0)
  line L0 (-55, -42.5) -> (-85, -42.5) projected
  line L1 (-170, -7.5) -> (-176.6721, -7.5) projected
  line L2 (-55, -42.5) -> (-176.6721, -42.5)
  line L3 (-176.6721, -42.5) -> (-176.6721, -7.5)
  line L4 (-176.6721, -7.5) -> (-55, -7.5)
  line L5 (-55, -7.5) -> (-55, -42.5)
  point P0 (0, 0)
  constraints: 8 end point, 2 parallel, 1 horizontal, 1 perpendicular
extrude "Extrusion39" cut sketch "Sketch51" against normal blind 10
sketch "Sketch52" plane through (0, 7.5, 0) normal (0, 1, 0) x (1, 0, 0)
  line L0 (-176.6721, -7.5) -> (-55, -7.5) construction
  line L1 (-55, -42.5) -> (-129.724, -42.5) construction
  line L2 (-129.724, -42.5) -> (-129.724, -7.5) construction
  line L3 (-129.724, -7.5) -> (-55, -7.5) construction
  line L4 (-55, -7.5) -> (-55, -42.5) construction
  line L5 (-129.724, -7.5) -> (-204.448, -7.5) construction
  line L6 (-204.448, -7.5) -> (-204.448, -42.5) construction
  line L7 (-204.448, -42.5) -> (-129.724, -42.5) construction
  line L8 (-129.724, -42.5) -> (-129.724, -7.5) construction
  line L9 (-204.448, -7.5) -> (-129.724, -42.5) construction
  line L10 (-204.448, -42.5) -> (-129.724, -7.5) construction
  line L11 (-55, -42.5) -> (-55, -7.5) construction
  line L12 (-129.724, -7.5) -> (-55, -42.5) construction
  line L13 (-55, -42.5) -> (-129.724, -42.5) construction
  line L14 (-55, -42.5) -> (-176.6721, -42.5) construction
  line L15 (-129.724, -42.5) -> (-55, -7.5) construction
  line L16 (-129.4259, -4.5997) -> (-206.8669, -40.8724)
  line L17 (-206.8669, -40.8724) -> (-204.7461, -45.4003)
  line L18 (-204.7461, -45.4003) -> (-127.3051, -9.1276)
  line L19 (-127.3051, -9.1276) -> (-129.4259, -4.5997)
  line L20 (-129.4259, -4.5997) -> (-204.7461, -45.4003) construction
  line L21 (-206.8669, -40.8724) -> (-127.3051, -9.1276) construction
  line L22 (-130.7844, -44.764) -> (-205.5084, -9.764)
  line L23 (-205.5084, -9.764) -> (-203.3876, -5.236)
  line L24 (-203.3876, -5.236) -> (-128.6636, -40.236)
  line L25 (-128.6636, -40.236) -> (-130.7844, -44.764)
  line L26 (-130.7844, -44.764) -> (-203.3876, -5.236) construction
  line L27 (-205.5084, -9.764) -> (-128.6636, -40.236) construction
  line L28 (-130.0221, -45.4003) -> (-52.5811, -9.1276)
  line L29 (-52.5811, -9.1276) -> (-54.7019, -4.5997)
  line L30 (-54.7019, -4.5997) -> (-132.1429, -40.8724)
  line L31 (-132.1429, -40.8724) -> (-130.0221, -45.4003)
  line L32 (-130.0221, -45.4003) -> (-54.7019, -4.5997) construction
  line L33 (-52.5811, -9.1276) -> (-132.1429, -40.8724) construction
  line L34 (-130.351, -5.219) -> (-52.3266, -40.219)
  line L35 (-52.3266, -40.219) -> (-54.373, -44.781)
  line L36 (-54.373, -44.781) -> (-132.3974, -9.781)
  line L37 (-132.3974, -9.781) -> (-130.351, -5.219)
  line L38 (-130.351, -5.219) -> (-54.373, -44.781) construction
  line L39 (-52.3266, -40.219) -> (-132.3974, -9.781) construction
  point P0 (0, 0)
  point P1 (-167.086, -25)
  point P2 (-167.086, -25)
  point P3 (-92.362, -25)
  point P4 (-92.362, -25)
  dimension "d233" = 74.724
  dimension "d234" = 74.724
  dimension "d235" = 85.515
  dimension "d236" = 5
  dimension "d237" = 5
  dimension "d238" = 85.515
  dimension "d239" = 5
  dimension "d240" = 85.515
  dimension "d241" = 5
  constraints: 74 end point, 13 parallel, 12 midpoint, 7 perpendicular, 2 horizontal, 2 point on line, 1 collinear
  measures "d233" distance of L2.end L3.end
  measures "d234" distance of L7.end L6.end
  measures "d235" distance of L16.start L16.end
  measures "d236" distance of L17.end L16.end
  measures "d237" distance of L22.end L23.end
  measures "d238" distance of L28.start L28.end
  measures "d239" distance of L29.end L28.end
  measures "d240" distance of L34.start L34.end
  measures "d241" distance of L34.end L35.end
extrude "Extrusion40" add sketch "Sketch52" against normal blind 2 contours L19 L34 L37 L36 L18 L24 L16 | L24 L18 L22 L16 | L16 L22 L23 L24 | L34 L30 L36 L18 L19 | L19 L18 L36 L37 L34 | L22 L18 L17 L16 | L24 L30 L31 L25 L22 L18 | L34 L28 L36 L30 | L30 L29 L28 L34 | L30 L36 L28 L31 L25 L24 | L24 L25 L31 L30 | L34 L35 L36 L28
fillet "Fillet9" radius 2 11 edges at (-167.086, 6.5, 27.7606) (-130.5088, 6.5, 10.6282) (-161.1921, 6.5, 25) (-123.8301, 6.5, 42.5) (-86.3633, 6.5, 24.9509) (-167.086, 6.5, 22.2394) (-129.724, 6.5, 39.7394) (-55, 6.5, 39.0197) (-92.3845, 6.5, 22.2499) (-92.3395, 6.5, 27.7501) (-55, 6.5, 10.2606)
fillet "Fillet10" radius 2 4 edges at (-135.6179, 6.5, 42.5) (-172.9799, 6.5, 25) (-135.6179, 6.5, 7.5) (-60.8939, 6.5, 7.5)
fillet "Fillet11" radius 2 2 edges at (-125.266, 6.5, 7.5) (-59.458, 6.5, 42.5)
fillet "Fillet12" radius 2 1 edges at (-98.3607, 6.5, 25.0491)
sketch "Sketch53" plane through (0, 7.5, 0) normal (0, 1, 0) x (1, 0, 0)
  line L0 (-19.425, 0) -> (-176.6721, 0) projected
  line L1 (-176.6721, 0) -> (-186.6721, 0)
  line L2 (-186.6721, 0) -> (-186.6721, -51.3376)
  line L3 (-186.6721, -51.3376) -> (-176.6721, -51.3376)
  line L4 (-176.6721, -51.3376) -> (-176.6721, 0)
  line L5 (-186.6721, -51.3376) -> (-210.4355, -51.3376)
  line L6 (-210.4355, -51.3376) -> (-210.4355, 0)
  line L7 (-210.4355, 0) -> (-186.6721, 0)
  line L8 (-186.6721, 0) -> (-186.6721, -51.3376)
  point P0 (0, 0)
  dimension "d248" = 10
  constraints: 16 end point, 4 parallel, 2 horizontal, 2 perpendicular, 1 point on line
  measures "d248" distance of L3.end L2.end
extrude "Extrusion41" cut sketch "Sketch53" against normal blind 2 contours L2 L5 L6 L7
sketch "Sketch54" plane through (0, 7.5, 0) normal (0, 1, 0) x (1, 0, 0)
  line L0 (-176.6721, -42.5) -> (-176.6721, -50) projected
  line L1 (-176.6721, -50) -> (-187.6003, -50)
  line L2 (-187.6003, -50) -> (-187.6003, 0)
  line L3 (-187.6003, 0) -> (-176.6721, 0)
  line L4 (-176.6721, 0) -> (-176.6721, -50)
  point P0 (0, 0)
  constraints: 8 end point, 2 parallel, 1 horizontal, 1 perpendicular
extrude "Extrusion42" cut sketch "Sketch54" against normal blind 1
sketch "Sketch55" plane through (0, 0, 44.3276) normal (1, 0, 0) x (0, 0, -1)
  point P0 (44.3276, 0)
sketch "Sketch56" plane through (0, 0, 0) normal (0, -1, 0) x (1, 0, 0)
  line L0 (-19.425, 0) -> (-176.6721, 0) projected
  line L1 (-186.6721, 7.5) -> (-166.6721, 7.5)
  line L2 (-166.6721, 7.5) -> (-166.6721, 0)
  line L3 (-166.6721, 0) -> (-186.6721, 0)
  line L4 (-186.6721, 0) -> (-186.6721, 7.5)
  line L5 (-176.6721, 0) -> (-176.6721, 7.5) projected
  line L6 (-186.6721, 7.5) -> (-166.6721, 0) construction
  line L7 (-166.6721, 7.5) -> (-186.6721, 0) construction
  point P0 (0, 0)
  point P1 (-176.6721, 3.75)
  dimension "d253" = 20
  constraints: 12 end point, 3 midpoint, 2 parallel, 1 horizontal, 1 perpendicular, 1 point on line
  measures "d253" distance of L2.end L3.end
extrude "Extrusion43" add sketch "Sketch56" along normal blind 1
sketch "Sketch57" plane through (0, 0, 44.3276) normal (1, 0, 0) x (0, 0, -1)
  circle A0 centre (-16.9224, 3.75) radius 3 projected
  circle A1 centre (-16.9224, 3.75) radius 3
  line L0 (-10.6724, -2) -> (-22.6724, -2) projected
  line L1 (-5.6724, 7.5) -> (-22.6724, 7.5) projected
  line L2 (-10.6724, -2) -> (-22.6724, -2)
  line L3 (-22.6724, -2) -> (-22.6724, 7.5)
  line L4 (-22.6724, 7.5) -> (-10.6724, 7.5)
  line L5 (-10.6724, 7.5) -> (-10.6724, -2)
  point P0 (44.3276, 0)
  constraints: 8 end point, 2 parallel, 1 centre point, 1 coincident, 1 horizontal, 1 perpendicular
extrude "Extrusion44" add sketch "Sketch57" along normal blind 0.5
body "Solid1"
